Autodesk Fusion 360 part; units mm, degrees
note: some values were not read from the file. Chosen so that the rebuilt part matches the saved one: which face or edge a step refers to. Set by a fixed rule: which sketch regions a step uses.
(part 3 of 4)
sketch "Sketch5 (5)" plane through (0, 24.0807, 0) normal (0, 1, 0) x (-1, 0, 0) in component "ButtonRed v5"
  circle A0 centre (80.5, -16.1) radius 2.1574
  circle A1 centre (80.5, 16.1) radius 2.1574
  circle A2 centre (-80.5, -16.1) radius 2.1574
  circle A3 centre (-80.5, 16.1) radius 2.1574
  line L0 (-81.5, -11.1) -> (-83.5, -11.1)
  line L1 (-83.5, -11.1) -> (-83.5, -19.1)
  line L2 (-83.5, -19.1) -> (-75.5, -19.1)
  line L3 (-75.5, -19.1) -> (-75.5, -17.1)
  line L4 (-75.5, -17.1) -> (-45.2, -17.1)
  line L5 (-45.2, -17.1) -> (-45.2, -19.1)
  line L6 (-45.2, -19.1) -> (-37.2, -19.1)
  line L7 (-37.2, -19.1) -> (-37.2, -17.1)
  line L8 (-37.2, -17.1) -> (-4, -17.1)
  line L9 (-4, -17.1) -> (-4, -19.1)
  line L10 (-4, -19.1) -> (4, -19.1)
  line L11 (4, -19.1) -> (4, -17.1)
  line L12 (4, -17.1) -> (37.2, -17.1)
  line L13 (37.2, -17.1) -> (37.2, -19.1)
  line L14 (37.2, -19.1) -> (45.2, -19.1)
  line L15 (45.2, -19.1) -> (45.2, -17.1)
  line L16 (45.2, -17.1) -> (75.5, -17.1)
  line L17 (75.5, -17.1) -> (75.5, -19.1)
  line L18 (75.5, -19.1) -> (83.5, -19.1)
  line L19 (83.5, -19.1) -> (83.5, -11.1)
  line L20 (83.5, -11.1) -> (81.5, -11.1)
  line L21 (81.5, -11.1) -> (81.5, 11.1)
  line L22 (81.5, 11.1) -> (83.5, 11.1)
  line L23 (83.5, 11.1) -> (83.5, 19.1)
  line L24 (83.5, 19.1) -> (75.5, 19.1)
  line L25 (75.5, 19.1) -> (75.5, 17.1)
  line L26 (75.5, 17.1) -> (45.2, 17.1)
  line L27 (45.2, 17.1) -> (45.2, 19.1)
  line L28 (45.2, 19.1) -> (37.2, 19.1)
  line L29 (37.2, 19.1) -> (37.2, 17.1)
  line L30 (37.2, 17.1) -> (4, 17.1)
  line L31 (4, 17.1) -> (4, 19.1)
  line L32 (4, 19.1) -> (-4, 19.1)
  line L33 (-4, 19.1) -> (-4, 17.1)
  line L34 (-4, 17.1) -> (-37.2, 17.1)
  line L35 (-37.2, 17.1) -> (-37.2, 19.1)
  line L36 (-37.2, 19.1) -> (-45.2, 19.1)
  line L37 (-45.2, 19.1) -> (-45.2, 17.1)
  line L38 (-45.2, 17.1) -> (-75.5, 17.1)
  line L39 (-75.5, 17.1) -> (-75.5, 19.1)
  line L40 (-75.5, 19.1) -> (-83.5, 19.1)
  line L41 (-83.5, 19.1) -> (-83.5, 11.1)
  line L42 (-83.5, 11.1) -> (-81.5, 11.1)
  line L43 (-81.5, 11.1) -> (-81.5, -11.1)
  line L44 (-1, -11.1) -> (-1, 11.1)
  line L45 (-1, 11.1) -> (1, 11.1)
  line L46 (1, 11.1) -> (1, -11.1)
  line L47 (1, -11.1) -> (-1, -11.1)
  line L48 (-42.2, -11.1) -> (-42.2, 11.1)
  line L49 (-42.2, 11.1) -> (-40.2, 11.1)
  line L50 (-40.2, 11.1) -> (-40.2, -11.1)
  line L51 (-40.2, -11.1) -> (-42.2, -11.1)
  circle A4 centre (-61.8, 12.9) radius 3.1
  circle A5 centre (-20.6, 12.9) radius 3.1
  circle A6 centre (36, 0) radius 3.1
  circle A7 centre (77.2, 0) radius 3.1
  circle A8 centre (61.8, -12.9) radius 3.1
  circle A9 centre (20.6, -12.9) radius 3.1
  circle A10 centre (-5.2, 0) radius 3.1
  circle A11 centre (-61.8, -12.9) radius 3.1
  circle A12 centre (-46.4, 0) radius 3.1
  circle A13 centre (-20.6, -12.9) radius 3.1
  circle A14 centre (20.6, 12.9) radius 3.1
  circle A15 centre (61.8, 12.9) radius 3.1
  circle A16 centre (46.4, 0) radius 3.1
  circle A17 centre (5.2, 0) radius 3.1
  circle A18 centre (-36, 0) radius 3.1
  circle A19 centre (-77.2, 0) radius 3.1
  line L52 (9.4, 8.7) -> (31.8, 8.7)
  line L53 (31.8, 8.7) -> (31.8, -8.7)
  line L54 (31.8, -8.7) -> (9.4, -8.7)
  line L55 (9.4, -8.7) -> (9.4, 8.7)
  line L56 (-31.8, 8.7) -> (-9.4, 8.7)
  line L57 (-9.4, 8.7) -> (-9.4, -8.7)
  line L58 (-9.4, -8.7) -> (-31.8, -8.7)
  line L59 (-31.8, -8.7) -> (-31.8, 8.7)
  line L60 (73, 8.7) -> (73, -8.7)
  line L61 (73, -8.7) -> (50.6, -8.7)
  line L62 (50.6, -8.7) -> (50.6, 8.7)
  line L63 (50.6, 8.7) -> (73, 8.7)
  line L64 (-73, 8.7) -> (-50.6, 8.7)
  line L65 (-50.6, 8.7) -> (-50.6, -8.7)
  line L66 (-50.6, -8.7) -> (-73, -8.7)
  line L67 (-73, -8.7) -> (-73, 8.7)
  line L68 (42.2, 11.1) -> (42.2, -11.1)
  line L69 (42.2, -11.1) -> (40.2, -11.1)
  line L70 (40.2, -11.1) -> (40.2, 11.1)
  line L71 (40.2, 11.1) -> (42.2, 11.1)
  circle A20 centre (20.6, 12.9) radius 3.1
  line L72 (-1, -11.1) -> (1, -11.1)
  line L73 (1, -11.1) -> (1, 11.1)
  line L74 (1, 11.1) -> (-1, 11.1)
  line L75 (-1, 11.1) -> (-1, -11.1)
  circle A21 centre (20.6, -12.9) radius 3.1
  line L76 (4, -19.1) -> (37.2, -19.1)
  line L77 (37.2, -19.1) -> (37.2, -17.1)
  line L78 (37.2, -17.1) -> (4, -17.1)
  line L79 (4, -17.1) -> (4, -19.1)
  line L80 (42.2, 11.1) -> (40.2, 11.1)
  line L81 (40.2, 11.1) -> (40.2, -11.1)
  line L82 (40.2, -11.1) -> (42.2, -11.1)
  line L83 (42.2, -11.1) -> (42.2, 11.1)
  line L84 (37.2, 19.1) -> (4, 19.1)
  line L85 (4, 19.1) -> (4, 17.1)
  line L86 (4, 17.1) -> (37.2, 17.1)
  line L87 (37.2, 17.1) -> (37.2, 19.1)
  line L88 (39.6, -16.8333) -> (1.6, -16.8333)
  line L89 (1.6, -16.8333) -> (1.6, 16.6667)
  line L90 (1.6, 16.6667) -> (39.6, 16.6667)
  line L91 (39.6, 16.6667) -> (39.6, -16.8333)
  line L92 (39.6, -16.8333) -> (1.6, 16.6667) construction
  line L93 (1.6, -16.8333) -> (39.6, 16.6667) construction
  point P0 (5.2, 0)
  point P1 (20.6, -12.9)
  point P2 (20.6, -0.0833)
  dimension "d849_2" = 38
  dimension "d850_2" = 33.5
  constraint perpendicular L88 L89
  constraint parallel L88 L90
  constraint parallel L89 L91
  constraint horizontal L88
  constraint coincident L92 P2
  constraint coincident L93 P2
  measures "d849_2" distance of L89.end L90.end
  measures "d850_2" distance of L88.end L89.end
extrude "Extrude5''''" [suppressed] in component "ButtonRed v5"
sketch "Sketch7 (4)" plane through (0, 24.0807, 0) normal (0, 1, 0) x (-1, 0, 0) in component "ButtonRed v5"
  circle A0 centre (20.6, -12.9) radius 3.1
  circle A1 centre (20.6, 12.9) radius 3.1
  circle A2 centre (5.2, 0) radius 3.1
  circle A3 centre (36, 0) radius 3.1
  line L0 (39.6, 16.6667) -> (1.6, 16.6667)
  line L1 (1.6, 16.6667) -> (1.6, -16.8333)
  line L2 (1.6, -16.8333) -> (39.6, -16.8333)
  line L3 (39.6, -16.8333) -> (39.6, 16.6667)
  line L4 (39.6, -16.8333) -> (1.6, -16.8333)
  line L5 (1.6, -16.8333) -> (1.6, 16.6667)
  line L6 (1.6, 16.6667) -> (39.6, 16.6667)
  line L7 (39.6, 16.6667) -> (39.6, -16.8333)
  dimension "d859_2" = 38
  constraint horizontal L4
  constraint vertical L5
  constraint horizontal L6
  constraint vertical L7
  constraint coincident L0.end L1.start
  constraint coincident L2.end L3.start
  measures "d859_2" distance of L2.end L1.end
extrude "Extrude7''" [suppressed] in component "ButtonRed v5"
sketch "Sketch8 (4)" plane through (0, 25.2807, 0) normal (0, 1, 0) x (-1, 0, 0) in component "ButtonRed v5"
  line L0 (39.6, 16.6667) -> (1.6, 16.6667)
  line L1 (1.6, 16.6667) -> (1.6, -16.8333)
  line L2 (1.6, -16.8333) -> (39.6, -16.8333)
  line L3 (39.6, -16.8333) -> (39.6, 16.6667)
  circle A0 centre (20.6, -0.0833) radius 14
  dimension "d862_2" = 19
  dimension "d863_2" = 16.75
  dimension "d864_2" = 28
  dimension "d865_2" = 38
  dimension "d866_2" = 33.5
  measures "d862_2" distance of L1 A0.centre
  measures "d863_2" distance of L0 A0.centre
  measures "d864_2" diameter of A0
  measures "d865_2" distance of L1.end L2.end
  measures "d866_2" distance of L0.start L2.end
extrude "Extrude8'''" [suppressed] in component "ButtonRed v5"
sketch "Sketch9 (4)" plane through (-1.6, 0, 0) normal (1, 0, 0) x (0, 0, -1) in component "ButtonRed v5"
  line L0 (-16.6667, 25.2807) -> (-16.6667, 22.2807)
  line L1 (-16.6667, 22.2807) -> (16.8333, 22.2807)
  line L2 (16.8333, 22.2807) -> (16.8333, 25.2807)
  line L3 (16.8333, 25.2807) -> (-16.6667, 25.2807)
other "Base Feature1''" in component "ButtonGreen v6"
sketch "Sketch1 (7)" plane through (0, 45, 0) normal (0, 1, 0) x (-1, 0, 0) in component "ButtonGreen v6"
  line L0 (-111.8498, 7.1011) -> (-111.8498, -10.2989)
  line L1 (-111.8498, -10.2989) -> (-134.2498, -10.2989)
  line L2 (-134.2498, -10.2989) -> (-134.2498, 7.1011)
  line L3 (-134.2498, 7.1011) -> (-111.8498, 7.1011)
  circle A0 centre (-138.4498, -1.5989) radius 3.1
  circle A1 centre (-123.0498, 11.3011) radius 3.1
  circle A2 centre (-123.0498, -14.4989) radius 3.1
  circle A3 centre (-107.6498, -1.5989) radius 3.1
  line L4 (-103.4498, -18.6989) -> (-103.4498, 15.5011)
  line L5 (-103.4498, 15.5011) -> (-142.6498, 15.5011)
  line L6 (-142.6498, 15.5011) -> (-142.6498, -18.6989)
  line L7 (-142.6498, -18.6989) -> (-103.4498, -18.6989)
  circle A4 centre (-138.4498, -1.5989) radius 3.1
  circle A5 centre (-123.0498, -14.4989) radius 3.1
  circle A6 centre (-107.6498, -1.5989) radius 3.1
  circle A7 centre (-123.0498, 11.3011) radius 3.1
  line L8 (-154.8498, 7.1011) -> (-154.8498, -10.2989)
  line L9 (-177.2498, -10.2989) -> (-177.2498, 7.1011)
  line L10 (-146.7095, 15.4507) -> (-185.4095, 15.5014)
  line L11 (-177.2498, 7.1011) -> (-154.8498, 7.1011)
  circle A8 centre (-166.0498, -14.4989) radius 3.1
  circle A9 centre (-181.4498, -1.5989) radius 3.1
  line L12 (-185.4095, 15.5014) -> (-185.4536, -18.1986)
  circle A10 centre (-181.4498, -1.5989) radius 3.1
  line L13 (-146.7537, -18.2493) -> (-146.7095, 15.4507)
  circle A11 centre (-166.0498, 11.3011) radius 3.1
  circle A12 centre (-166.0498, 11.3011) radius 3.1
  line L14 (-154.8498, -10.2989) -> (-177.2498, -10.2989)
  circle A13 centre (-150.6498, -1.5989) radius 3.1
  circle A14 centre (-150.6498, -1.5989) radius 3.1
  line L15 (-185.4536, -18.1986) -> (-146.7537, -18.2493)
  circle A15 centre (-166.0498, -14.4989) radius 3.1
  arc A16 (86.5, -27.2432) -> (86.5, -22.3568) centre (88.5, -24.8) ccw
  arc A17 (-86.5, -22.3568) -> (-86.5, -27.2432) centre (-88.5, -24.8) ccw
  line L16 (86.5, 29) -> (-86.5, 29)
  line L17 (-86.5, 29) -> (-86.5, 27.2432)
  line L18 (-86.5, -29) -> (86.5, -29)
  line L19 (86.5, -29) -> (86.5, -27.2432)
  arc A18 (86.5, 22.3568) -> (86.5, 27.2432) centre (88.5, 24.8) ccw
  arc A19 (-86.5, 27.2432) -> (-86.5, 22.3568) centre (-88.5, 24.8) ccw
  line L20 (-86.5, 22.3568) -> (-86.5, -22.3568)
  line L21 (-86.5, -27.2432) -> (-86.5, -29)
  line L22 (86.5, -22.3568) -> (86.5, 22.3568)
  line L23 (86.5, 27.2432) -> (86.5, 29)
  dimension "d623_1" = 39.2
  dimension "d624_1" = 38.7
  dimension "d625_1" = 33.7
  dimension "d921_1" = 0
  dimension "d922_1" = 0
  dimension "d923_1" = 0
  dimension "d924_1" = 0
  constraint perpendicular L12 L15
  constraint parallel L10 L15
  constraint parallel L12 L13
  measures "d623_1" distance of L4.start L6.end
  measures "d624_1" distance of L13.start L12.end
  measures "d625_1" vertical distance of L10.end L12.end
extrude "Extrude1'''''" [suppressed] in component "ButtonGreen v6"
sketch "Sketch2 (6)" plane through (0, 45, 0) normal (0, 1, 0) x (-1, 0, 0) in component "ButtonGreen v6"
  line L0 (-142.6498, -18.6989) -> (-103.4498, -18.6989)
  line L1 (-103.4498, -18.6989) -> (-103.4498, 15.5011)
  line L2 (-103.4498, 15.5011) -> (-142.6498, 15.5011)
  line L3 (-142.6498, 15.5011) -> (-142.6498, -18.6989)
extrude "Extrude2''''''" [suppressed] in component "ButtonGreen v6"
sketch "Sketch3 (6)" plane through (0, 49.8, 0) normal (0, 1, 0) x (-1, 0, 0) in component "ButtonGreen v6"
  line L0 (-142.6498, 15.5011) -> (-142.6498, -18.6989)
  line L1 (-142.6498, -18.6989) -> (-103.4498, -18.6989)
  line L2 (-103.4498, -18.6989) -> (-103.4498, 15.5011)
  line L3 (-103.4498, 15.5011) -> (-142.6498, 15.5011)
  circle A0 centre (-123.0498, -1.5989) radius 14
  dimension "d616_1" = 28
  dimension "d617_1" = 17.1
  dimension "d618_1" = 34.2
  dimension "d619_1" = 39.2
  dimension "d620_1" = 19.6
  measures "d616_1" diameter of A0
  measures "d617_1" distance of L1 A0.centre
  measures "d618_1" distance of L1 L3
  measures "d619_1" distance of L0 L2
  measures "d620_1" distance of L2 A0.centre
extrude "Extrude3'''''" [suppressed] in component "ButtonGreen v6"
sketch "Sketch4 (6)" plane through (0, 49.8, 0) normal (0, 1, 0) x (-1, 0, 0) in component "ButtonGreen v6"
  circle A0 centre (-123.0498, -1.5989) radius 14
  line L0 (-142.6498, 15.5011) -> (-142.6498, -18.6989)
  line L1 (-142.6498, -18.6989) -> (-103.4498, -18.6989)
  line L2 (-103.4498, -18.6989) -> (-103.4498, 15.5011)
  line L3 (-103.4498, 15.5011) -> (-142.6498, 15.5011)
  line L4 (-103.9498, 15.0011) -> (-142.1498, 15.0011)
  line L5 (-142.1498, 15.0011) -> (-142.1498, -18.1989)
  line L6 (-142.1498, -18.1989) -> (-103.9498, -18.1989)
  line L7 (-103.9498, -18.1989) -> (-103.9498, 15.0011)
  dimension "d627_1" = -0.5
extrude "Extrude4'''''" [suppressed] in component "ButtonGreen v6"
sketch "Sketch10 (4)" plane through (0, 37.0807, 0) normal (0, 1, 0) x (-1, 0, 0) in component "ButtonGreen v6"
  circle A0 centre (80.75, -16) radius 2.1574
  circle A1 centre (80.75, 16.2) radius 2.1574
  circle A2 centre (-80.25, -16) radius 2.1574
  circle A3 centre (-80.25, 16.2) radius 2.1574
  line L0 (-81.25, -11) -> (-83.25, -11)
  line L1 (-83.25, -11) -> (-83.25, -19)
  line L2 (-83.25, -19) -> (-75.25, -19)
  line L3 (-75.25, -19) -> (-75.25, -17)
  line L4 (-75.25, -17) -> (-44.95, -17)
  line L5 (-44.95, -17) -> (-44.95, -19)
  line L6 (-44.95, -19) -> (-36.95, -19)
  line L7 (-36.95, -19) -> (-36.95, -17)
  line L8 (-36.95, -17) -> (-3.75, -17)
  line L9 (-3.75, -17) -> (-3.75, -19)
  line L10 (-3.75, -19) -> (4.25, -19)
  line L11 (4.25, -19) -> (4.25, -17)
  line L12 (4.25, -17) -> (37.45, -17)
  line L13 (37.45, -17) -> (37.45, -19)
  line L14 (37.45, -19) -> (45.45, -19)
  line L15 (45.45, -19) -> (45.45, -17)
  line L16 (45.45, -17) -> (75.75, -17)
  line L17 (75.75, -17) -> (75.75, -19)
  line L18 (75.75, -19) -> (83.75, -19)
  line L19 (83.75, -19) -> (83.75, -11)
  line L20 (83.75, -11) -> (81.75, -11)
  line L21 (81.75, -11) -> (81.75, 11.2)
  line L22 (81.75, 11.2) -> (83.75, 11.2)
  line L23 (83.75, 11.2) -> (83.75, 19.2)
  line L24 (83.75, 19.2) -> (75.75, 19.2)
  line L25 (75.75, 19.2) -> (75.75, 17.2)
  line L26 (75.75, 17.2) -> (45.45, 17.2)
  line L27 (45.45, 17.2) -> (45.45, 19.2)
  line L28 (45.45, 19.2) -> (37.45, 19.2)
  line L29 (37.45, 19.2) -> (37.45, 17.2)
  line L30 (37.45, 17.2) -> (4.25, 17.2)
  line L31 (4.25, 17.2) -> (4.25, 19.2)
  line L32 (4.25, 19.2) -> (-3.75, 19.2)
  line L33 (-3.75, 19.2) -> (-3.75, 17.2)
  line L34 (-3.75, 17.2) -> (-36.95, 17.2)
  line L35 (-36.95, 17.2) -> (-36.95, 19.2)
  line L36 (-36.95, 19.2) -> (-44.95, 19.2)
  line L37 (-44.95, 19.2) -> (-44.95, 17.2)
  line L38 (-44.95, 17.2) -> (-75.25, 17.2)
  line L39 (-75.25, 17.2) -> (-75.25, 19.2)
  line L40 (-75.25, 19.2) -> (-83.25, 19.2)
  line L41 (-83.25, 19.2) -> (-83.25, 11.2)
  line L42 (-83.25, 11.2) -> (-81.25, 11.2)
  line L43 (-81.25, 11.2) -> (-81.25, -11)
  line L44 (-0.75, -11) -> (-0.75, 11.2)
  line L45 (-0.75, 11.2) -> (1.25, 11.2)
  line L46 (1.25, 11.2) -> (1.25, -11)
  line L47 (1.25, -11) -> (-0.75, -11)
  line L48 (-41.95, -11) -> (-41.95, 11.2)
  line L49 (-41.95, 11.2) -> (-39.95, 11.2)
  line L50 (-39.95, 11.2) -> (-39.95, -11)
  line L51 (-39.95, -11) -> (-41.95, -11)
  circle A4 centre (-61.55, 13) radius 3.1
  circle A5 centre (-20.35, 13) radius 3.1
  circle A6 centre (36.25, 0.1) radius 3.1
  circle A7 centre (77.45, 0.1) radius 3.1
  circle A8 centre (62.05, -12.8) radius 3.1
  circle A9 centre (20.85, -12.8) radius 3.1
  circle A10 centre (-4.95, 0.1) radius 3.1
  circle A11 centre (-61.55, -12.8) radius 3.1
  circle A12 centre (-46.15, 0.1) radius 3.1
  circle A13 centre (-20.35, -12.8) radius 3.1
  circle A14 centre (20.85, 13) radius 3.1
  circle A15 centre (62.05, 13) radius 3.1
  circle A16 centre (46.65, 0.1) radius 3.1
  circle A17 centre (5.45, 0.1) radius 3.1
  circle A18 centre (-35.75, 0.1) radius 3.1
  circle A19 centre (-76.95, 0.1) radius 3.1
  line L52 (9.65, 8.8) -> (32.05, 8.8)
  line L53 (32.05, 8.8) -> (32.05, -8.6)
  line L54 (32.05, -8.6) -> (9.65, -8.6)
  line L55 (9.65, -8.6) -> (9.65, 8.8)
  line L56 (-31.55, 8.8) -> (-9.15, 8.8)
  line L57 (-9.15, 8.8) -> (-9.15, -8.6)
  line L58 (-9.15, -8.6) -> (-31.55, -8.6)
  line L59 (-31.55, -8.6) -> (-31.55, 8.8)
  line L60 (73.25, 8.8) -> (73.25, -8.6)
  line L61 (73.25, -8.6) -> (50.85, -8.6)
  line L62 (50.85, -8.6) -> (50.85, 8.8)
  line L63 (50.85, 8.8) -> (73.25, 8.8)
  line L64 (-72.75, 8.8) -> (-50.35, 8.8)
  line L65 (-50.35, 8.8) -> (-50.35, -8.6)
  line L66 (-50.35, -8.6) -> (-72.75, -8.6)
  line L67 (-72.75, -8.6) -> (-72.75, 8.8)
  line L68 (42.45, 11.2) -> (42.45, -11)
  line L69 (42.45, -11) -> (40.45, -11)
  line L70 (40.45, -11) -> (40.45, 11.2)
  line L71 (40.45, 11.2) -> (42.45, 11.2)
  circle A20 centre (62.05, 13) radius 3.1
  circle A21 centre (46.65, 0.1) radius 3.1
  circle A22 centre (62.05, -12.8) radius 3.1
  circle A23 centre (77.45, 0.1) radius 3.1
sketch "Sketch5 (6)" plane through (0, 24.0807, 0) normal (0, 1, 0) x (-1, 0, 0) in component "ButtonGreen v6"
  circle A0 centre (80.5, -16.1) radius 2.1574
  circle A1 centre (80.5, 16.1) radius 2.1574
  circle A2 centre (-80.5, -16.1) radius 2.1574
  circle A3 centre (-80.5, 16.1) radius 2.1574
  line L0 (-81.5, -11.1) -> (-83.5, -11.1)
  line L1 (-83.5, -11.1) -> (-83.5, -19.1)
  line L2 (-83.5, -19.1) -> (-75.5, -19.1)
  line L3 (-75.5, -19.1) -> (-75.5, -17.1)
  line L4 (-75.5, -17.1) -> (-45.2, -17.1)
  line L5 (-45.2, -17.1) -> (-45.2, -19.1)
  line L6 (-45.2, -19.1) -> (-37.2, -19.1)
  line L7 (-37.2, -19.1) -> (-37.2, -17.1)
  line L8 (-37.2, -17.1) -> (-4, -17.1)
  line L9 (-4, -17.1) -> (-4, -19.1)
  line L10 (-4, -19.1) -> (4, -19.1)
  line L11 (4, -19.1) -> (4, -17.1)
  line L12 (4, -17.1) -> (37.2, -17.1)
  line L13 (37.2, -17.1) -> (37.2, -19.1)
  line L14 (37.2, -19.1) -> (45.2, -19.1)
  line L15 (45.2, -19.1) -> (45.2, -17.1)
  line L16 (45.2, -17.1) -> (75.5, -17.1)
  line L17 (75.5, -17.1) -> (75.5, -19.1)
  line L18 (75.5, -19.1) -> (83.5, -19.1)
  line L19 (83.5, -19.1) -> (83.5, -11.1)
  line L20 (83.5, -11.1) -> (81.5, -11.1)
  line L21 (81.5, -11.1) -> (81.5, 11.1)
  line L22 (81.5, 11.1) -> (83.5, 11.1)
  line L23 (83.5, 11.1) -> (83.5, 19.1)
  line L24 (83.5, 19.1) -> (75.5, 19.1)
  line L25 (75.5, 19.1) -> (75.5, 17.1)
  line L26 (75.5, 17.1) -> (45.2, 17.1)
  line L27 (45.2, 17.1) -> (45.2, 19.1)
  line L28 (45.2, 19.1) -> (37.2, 19.1)
  line L29 (37.2, 19.1) -> (37.2, 17.1)
  line L30 (37.2, 17.1) -> (4, 17.1)
  line L31 (4, 17.1) -> (4, 19.1)
  line L32 (4, 19.1) -> (-4, 19.1)
  line L33 (-4, 19.1) -> (-4, 17.1)
  line L34 (-4, 17.1) -> (-37.2, 17.1)
  line L35 (-37.2, 17.1) -> (-37.2, 19.1)
  line L36 (-37.2, 19.1) -> (-45.2, 19.1)
  line L37 (-45.2, 19.1) -> (-45.2, 17.1)
  line L38 (-45.2, 17.1) -> (-75.5, 17.1)
  line L39 (-75.5, 17.1) -> (-75.5, 19.1)
  line L40 (-75.5, 19.1) -> (-83.5, 19.1)
  line L41 (-83.5, 19.1) -> (-83.5, 11.1)
  line L42 (-83.5, 11.1) -> (-81.5, 11.1)
  line L43 (-81.5, 11.1) -> (-81.5, -11.1)
  line L44 (-1, -11.1) -> (-1, 11.1)
  line L45 (-1, 11.1) -> (1, 11.1)
  line L46 (1, 11.1) -> (1, -11.1)
  line L47 (1, -11.1) -> (-1, -11.1)
  line L48 (-42.2, -11.1) -> (-42.2, 11.1)
  line L49 (-42.2, 11.1) -> (-40.2, 11.1)
  line L50 (-40.2, 11.1) -> (-40.2, -11.1)
  line L51 (-40.2, -11.1) -> (-42.2, -11.1)
  circle A4 centre (-61.8, 12.9) radius 3.1
  circle A5 centre (-20.6, 12.9) radius 3.1
  circle A6 centre (36, 0) radius 3.1
  circle A7 centre (77.2, 0) radius 3.1
  circle A8 centre (61.8, -12.9) radius 3.1
  circle A9 centre (20.6, -12.9) radius 3.1
  circle A10 centre (-5.2, 0) radius 3.1
  circle A11 centre (-61.8, -12.9) radius 3.1
  circle A12 centre (-46.4, 0) radius 3.1
  circle A13 centre (-20.6, -12.9) radius 3.1
  circle A14 centre (20.6, 12.9) radius 3.1
  circle A15 centre (61.8, 12.9) radius 3.1
  circle A16 centre (46.4, 0) radius 3.1
  circle A17 centre (5.2, 0) radius 3.1
  circle A18 centre (-36, 0) radius 3.1
  circle A19 centre (-77.2, 0) radius 3.1
  line L52 (9.4, 8.7) -> (31.8, 8.7)
  line L53 (31.8, 8.7) -> (31.8, -8.7)
  line L54 (31.8, -8.7) -> (9.4, -8.7)
  line L55 (9.4, -8.7) -> (9.4, 8.7)
  line L56 (-31.8, 8.7) -> (-9.4, 8.7)
  line L57 (-9.4, 8.7) -> (-9.4, -8.7)
  line L58 (-9.4, -8.7) -> (-31.8, -8.7)
  line L59 (-31.8, -8.7) -> (-31.8, 8.7)
  line L60 (73, 8.7) -> (73, -8.7)
  line L61 (73, -8.7) -> (50.6, -8.7)
  line L62 (50.6, -8.7) -> (50.6, 8.7)
  line L63 (50.6, 8.7) -> (73, 8.7)
  line L64 (-73, 8.7) -> (-50.6, 8.7)
  line L65 (-50.6, 8.7) -> (-50.6, -8.7)
  line L66 (-50.6, -8.7) -> (-73, -8.7)
  line L67 (-73, -8.7) -> (-73, 8.7)
  line L68 (42.2, 11.1) -> (42.2, -11.1)
  line L69 (42.2, -11.1) -> (40.2, -11.1)
  line L70 (40.2, -11.1) -> (40.2, 11.1)
  line L71 (40.2, 11.1) -> (42.2, 11.1)
  circle A20 centre (20.6, 12.9) radius 3.1
  line L72 (-1, -11.1) -> (1, -11.1)
  line L73 (1, -11.1) -> (1, 11.1)
  line L74 (1, 11.1) -> (-1, 11.1)
  line L75 (-1, 11.1) -> (-1, -11.1)
  circle A21 centre (20.6, -12.9) radius 3.1
  line L76 (4, -19.1) -> (37.2, -19.1)
  line L77 (37.2, -19.1) -> (37.2, -17.1)
  line L78 (37.2, -17.1) -> (4, -17.1)
  line L79 (4, -17.1) -> (4, -19.1)
  line L80 (42.2, 11.1) -> (40.2, 11.1)
  line L81 (40.2, 11.1) -> (40.2, -11.1)
  line L82 (40.2, -11.1) -> (42.2, -11.1)
  line L83 (42.2, -11.1) -> (42.2, 11.1)
  line L84 (37.2, 19.1) -> (4, 19.1)
  line L85 (4, 19.1) -> (4, 17.1)
  line L86 (4, 17.1) -> (37.2, 17.1)
  line L87 (37.2, 17.1) -> (37.2, 19.1)
  line L88 (39.6, -16.8333) -> (1.6, -16.8333)
  line L89 (1.6, -16.8333) -> (1.6, 16.6667)
  line L90 (1.6, 16.6667) -> (39.6, 16.6667)
  line L91 (39.6, 16.6667) -> (39.6, -16.8333)
  line L92 (39.6, -16.8333) -> (1.6, 16.6667) construction
  line L93 (1.6, -16.8333) -> (39.6, 16.6667) construction
  point P0 (5.2, 0)
  point P1 (20.6, -12.9)
  point P2 (20.6, -0.0833)
  dimension "d849_1" = 38
  dimension "d850_1" = 33.5
  constraint perpendicular L88 L89
  constraint parallel L88 L90
  constraint parallel L89 L91
  constraint horizontal L88
  constraint coincident L92 P2
  constraint coincident L93 P2
  measures "d849_1" distance of L89.end L90.end
  measures "d850_1" distance of L88.end L89.end
extrude "Extrude5'''''" [suppressed] in component "ButtonGreen v6"
sketch "Sketch7 (5)" plane through (0, 24.0807, 0) normal (0, 1, 0) x (-1, 0, 0) in component "ButtonGreen v6"
  circle A0 centre (20.6, -12.9) radius 3.1
  circle A1 centre (20.6, 12.9) radius 3.1
  circle A2 centre (5.2, 0) radius 3.1
  circle A3 centre (36, 0) radius 3.1
  line L0 (39.6, 16.6667) -> (1.6, 16.6667)
  line L1 (1.6, 16.6667) -> (1.6, -16.8333)
  line L2 (1.6, -16.8333) -> (39.6, -16.8333)
  line L3 (39.6, -16.8333) -> (39.6, 16.6667)
  line L4 (39.6, -16.8333) -> (1.6, -16.8333)
  line L5 (1.6, -16.8333) -> (1.6, 16.6667)
  line L6 (1.6, 16.6667) -> (39.6, 16.6667)
  line L7 (39.6, 16.6667) -> (39.6, -16.8333)
  dimension "d859_1" = 38
  constraint horizontal L4
  constraint vertical L5
  constraint horizontal L6
  constraint vertical L7
  constraint coincident L0.end L1.start
  constraint coincident L2.end L3.start
  measures "d859_1" distance of L2.end L1.end
extrude "Extrude7'''" [suppressed] in component "ButtonGreen v6"
sketch "Sketch8 (5)" plane through (0, 25.2807, 0) normal (0, 1, 0) x (-1, 0, 0) in component "ButtonGreen v6"
  line L0 (39.6, 16.6667) -> (1.6, 16.6667)
  line L1 (1.6, 16.6667) -> (1.6, -16.8333)
  line L2 (1.6, -16.8333) -> (39.6, -16.8333)
  line L3 (39.6, -16.8333) -> (39.6, 16.6667)
  circle A0 centre (20.6, -0.0833) radius 14
  dimension "d862_1" = 19
  dimension "d863_1" = 16.75
  dimension "d864_1" = 28
  dimension "d865_1" = 38
  dimension "d866_1" = 33.5
  measures "d862_1" distance of L1 A0.centre
  measures "d863_1" distance of L0 A0.centre
  measures "d864_1" diameter of A0
  measures "d865_1" distance of L1.end L2.end
  measures "d866_1" distance of L0.start L2.end
extrude "Extrude8''''" [suppressed] in component "ButtonGreen v6"
sketch "Sketch9 (5)" plane through (-1.6, 0, 0) normal (1, 0, 0) x (0, 0, -1) in component "ButtonGreen v6"
  line L0 (-16.6667, 25.2807) -> (-16.6667, 22.2807)
  line L1 (-16.6667, 22.2807) -> (16.8333, 22.2807)
  line L2 (16.8333, 22.2807) -> (16.8333, 25.2807)
  line L3 (16.8333, 25.2807) -> (-16.6667, 25.2807)
move_body "Move1" [suppressed] in component "Lid"
move_body "Move2" [suppressed] in component "Lid"
sketch "Sketch3 (7)" plane through (2.9698, 38.25, 1.2374) normal (0, 1, 0) x (-1, 0, 0) in component "Lid"
  line L0 (-61.7802, 11.7626) -> (125.7198, 11.7626)
  line L1 (125.7198, 11.7626) -> (125.7198, 69.7626)
  line L2 (-61.7802, 69.7626) -> (-61.7802, 11.7626)
  circle A0 centre (120.7198, 15.9626) radius 2
  circle A1 centre (120.7198, 65.5626) radius 2
  circle A2 centre (-56.7802, 15.9626) radius 2
  circle A3 centre (-56.7802, 65.5626) radius 2
  line L3 (125.7198, 69.7626) -> (-61.7802, 69.7626)
  dimension "d1030" = 4
  dimension "d1031" = 4.2
  dimension "d1033" = 187.5
  dimension "d1034" = 5
  dimension "d1035" = 5
  dimension "d1036" = 5
  dimension "d1037" = 4.2
  dimension "d1039" = 5
  constraint equal A0 A1
  constraint equal A0 A2
  constraint equal A0 A3
  measures "d1030" diameter of A0
  measures "d1031" distance of L0 A0.centre
  measures "d1033" distance of L0.start L0.end
  measures "d1034" distance of L1 A0.centre
  measures "d1035" distance of L1 A1.centre
  measures "d1036" distance of L2 A2.centre
  measures "d1037" distance of L0 A2.centre
  measures "d1039" distance of L2 A3.centre
extrude "Extrude3''''''" [suppressed] in component "Lid"
sketch "Sketch4 (7)" plane through (0, 38.25, 0) normal (0, 1, 0) x (-1, 0, 0) in component "Lid"
  line L0 (-64.75, 13) -> (122.75, 13)
  line L1 (122.75, 13) -> (122.75, 71)
  line L2 (-64.75, 71) -> (-64.75, 13)
  circle A0 centre (90.75, 43) radius 14.6
  line L3 (29, -29.0713) -> (29, 92.7233) construction
  line L4 (122.75, 71) -> (-64.75, 71)
  line L5 (-109.5632, 43) -> (-107.2358, 43)
  line L6 (-107.2358, 43) -> (154.5479, 43) construction
  circle A1 centre (49.55, 43) radius 14.6
  circle A2 centre (8.35, 43) radius 14.6
  circle A3 centre (-32.85, 43) radius 14.6
  circle A4 centre (117.75, 66.8) radius 2
  circle A5 centre (-59.75, 17.2) radius 2
  circle A6 centre (117.75, 17.2) radius 2
  circle A7 centre (-59.75, 66.8) radius 2
  line L7 (122.75, 71) -> (-64.75, 71)
  point P0 (29.9318, 42.6875)
  dimension "d1045" = 58
  dimension "d1053" = 29.2
  dimension "d1060" = 93.75
  dimension "d1061" = 187.5
  dimension "d1062" = 58
  dimension "d1064" = 30
  dimension "d1069" = 41.2
  dimension "d1070" = 41.2
  dimension "d1071" = 41.2
  dimension "d1085" = 32
  constraint vertical L3
  constraint horizontal L5
  constraint equal A0 A1
  constraint equal A1 A2
  constraint equal A2 A3
  constraint coincident A0.centre L6
  measures "d1045" distance of L0.start L2.start
  measures "d1053" diameter of A0
  measures "d1060" distance of L2 L3
  measures "d1061" distance of L1.end L2.start
  measures "d1062" distance of L0.start L2.start
  measures "d1064" distance of L0 L6
  measures "d1069" distance of A0.centre A1.centre
  measures "d1070" distance of A1.centre A2.centre
  measures "d1071" distance of A2.centre A3.centre
  measures "d1085" distance of L1 A0.centre
extrude "Extrude4''''''" [suppressed] in component "Lid"
sketch "Sketch16" plane through (0, 15, 0) normal (0, 1, 0) x (-1, 0, 0) in component "Button Base"
  line L0 (-4, 19.1) -> (-37.2, 19.1)
  line L1 (-37.2, 19.1) -> (-37.2, 17.1)
  line L2 (-37.2, 17.1) -> (-4, 17.1)
  line L3 (-4, 17.1) -> (-4, 19.1)
sketch "Sketch17" plane through (0, 0, 17.1) normal (0, 0, -1) x (-1, 0, 0) in component "Button Base"
  line L0 (-37.2, 7) -> (-4, 7)
  line L1 (-4, 7) -> (-4, 15)
  line L2 (-4, 15) -> (-37.2, 15)
  line L3 (-37.2, 15) -> (-37.2, 7)
ref_plane "WorkPlane3" through (40.2, 11, 0) normal (-1, 0, 0) x (0, 0, 1) in component "Button Base"
moveface "MoveFace1" [suppressed] in component "Button Base"
move_body "Move1'" [suppressed] in component "Button Base"
move_body "Move2'" [suppressed] in component "Button Base"
move_body "Move3" [suppressed] in component "Box"
move_body "Move3'" [suppressed] in component "Button Base"
ref_plane "WorkPlane1" through (-113.0665, 43.4789, -26.3874) normal (-1, 0, 0) x (0, 0, -1) in component "Component''"
sketch "Sketch4 (8)" plane through (0, 0, -66.2581) normal (0, 0, -1) x (-1, 0, 0)
  line L0 (21.2628, 41.0959) -> (194.7628, 41.0959)
  line L1 (194.7628, 41.0959) -> (194.7628, 74.0959)
  line L2 (194.7628, 74.0959) -> (21.2628, 74.0959)
  line L3 (21.2628, 74.0959) -> (21.2628, 41.0959)
sketch "Sketch8 (6)" plane through (0, 38.25, 0) normal (0, 1, 0) x (-1, 0, 0) in component "Lid"
  circle A0 centre (54.55, -2) radius 14.6
  circle A1 centre (13.35, -2) radius 14.6
  circle A2 centre (95.75, -2) radius 14.6
  circle A3 centre (-27.85, -2) radius 14.6
  line L0 (-59.75, -32) -> (127.75, -32)
  line L1 (127.75, -32) -> (127.75, 26)
  line L2 (-59.75, 26) -> (-59.75, -32)
  circle A4 centre (122.75, 21.8) radius 2
  circle A5 centre (-54.75, -27.8) radius 2
  circle A6 centre (122.75, -27.8) radius 2
  circle A7 centre (-54.75, 21.8) radius 2
  line L3 (127.75, 26) -> (-59.75, 26)
sketch "Sketch9 (6)" plane through (0, 38.25, 0) normal (0, 1, 0) x (-1, 0, 0) in component "Lid"
sketch "Sketch1 (8)" plane through (-190, 0, 2.6126) normal (0, 0, 1) x (1, 0, 0) in component "Component''"
  line L0 (150.6835, 28.4789) -> (-6.8165, 28.4789)
  line L1 (-6.8165, 58.4789) -> (-9.8165, 58.4789)
  line L2 (-9.8165, 58.4789) -> (-9.8165, 25.4789)
  line L3 (-9.8165, 25.4789) -> (163.6835, 25.4789)
  line L4 (-6.8165, 28.4789) -> (-6.8165, 20)
  line L5 (-6.8165, 20) -> (14.8335, 20)
  line L6 (14.8335, 20) -> (76.9209, 20)
  line L7 (76.9209, 20) -> (76.9209, 68.6959)
  line L8 (76.9209, 68.6959) -> (14.8335, 68.6959)
  line L9 (14.8335, 68.6959) -> (14.8335, 20)
  line L10 (163.6835, 25.4789) -> (163.6835, 58.4789)
  line L11 (163.6835, 58.4789) -> (150.6835, 58.4789)
  line L12 (150.6835, 58.4789) -> (150.6835, 28.4789)
  line L13 (-6.8165, 28.4789) -> (-6.8165, 58.4789)
  dimension "d1323" = 21.65
  constraint coincident L0.end L4.start
  constraint perpendicular L3 L4
  constraint perpendicular L4 L5
  constraint horizontal L6
  constraint vertical L7
  constraint horizontal L8
  constraint vertical L9
  measures "d1323" distance of L4.end L5.end
sketch "Sketch2 (7)" plane through (-190, 0, 2.6126) normal (0, 0, 1) x (1, 0, 0) in component "Component''"
  line L0 (-9.8165, 25.4789) -> (163.6835, 25.4789)
  line L1 (163.6835, 25.4789) -> (163.6835, 58.4789)
  line L2 (-6.8165, 58.4789) -> (-9.8165, 58.4789)
  line L3 (150.6835, 28.4789) -> (-6.8165, 28.4789)
  line L4 (150.6835, 28.4789) -> (128.5335, 28.4789)
  line L5 (128.5335, 28.4789) -> (128.5335, 68)
  line L6 (128.5335, 68) -> (60, 68)
  line L7 (60, 68) -> (60, 24.8783)
  line L8 (60, 24.8783) -> (128.5335, 24.8783)
  line L9 (128.5335, 24.8783) -> (128.5335, 28.4789)
  line L10 (-9.8165, 58.4789) -> (-9.8165, 25.4789)
  line L11 (163.6835, 58.4789) -> (150.6835, 58.4789)
  line L12 (150.6835, 58.4789) -> (150.6835, 28.4789)
  line L13 (-6.8165, 28.4789) -> (-6.8165, 58.4789)
  dimension "d1328" = 22.15
  constraint coincident L3.start L4.start
  constraint perpendicular L4 L5
  constraint perpendicular L5 L6
  constraint perpendicular L6 L7
  constraint perpendicular L7 L8
  constraint perpendicular L8 L9
  measures "d1328" distance of L3.start L4.end
sketch "Sketch3 (8)" plane through (-190, 0, 2.6126) normal (0, 0, 1) x (1, 0, 0) in component "Component''"
  line L0 (150.6835, 28.4789) -> (-6.8165, 28.4789)
  line L1 (-6.8165, 58.4789) -> (-9.8165, 58.4789)
  line L2 (-9.8165, 58.4789) -> (-9.8165, 25.4789)
  line L3 (-9.8165, 25.4789) -> (163.6835, 25.4789)
  line L4 (163.6835, 25.4789) -> (163.6835, 58.4789)
  line L5 (163.6835, 58.4789) -> (150.6835, 58.4789)
  line L6 (150.6835, 58.4789) -> (150.6835, 28.4789)
  line L7 (-6.8165, 28.4789) -> (-6.8165, 58.4789)
sketch "Sketch5 (7)" plane through (0, 0, 47.6126) normal (0, 0, 1) x (1, 0, 0) in component "Component''"
  line L0 (36.9372, 44.0959) -> (14.7872, 44.0959)
  line L1 (-1.8165, 28.4789) -> (-1.8165, 58.4789)
  line L2 (-1.8165, 58.4789) -> (-4.8165, 58.4789)
  line L3 (-4.8165, 58.4789) -> (-4.8165, 25.4789)
  line L4 (14.7872, 41.0959) -> (39.9372, 41.0959)
  line L5 (39.9372, 41.0959) -> (39.9372, 74.0959)
  line L6 (39.9372, 74.0959) -> (36.9372, 74.0959)
  line L7 (36.9372, 74.0959) -> (36.9372, 44.0959)
  line L8 (14.7872, 44.0959) -> (14.7872, 41.0959)
  line L9 (19.8335, 25.4789) -> (19.8335, 28.4789)
  line L10 (19.8335, 28.4789) -> (-1.8165, 28.4789)
  line L11 (-4.8165, 25.4789) -> (19.8335, 25.4789)
split "Split1" [suppressed] in component "Lid"
sketch "Sketch5 (8)" plane through (0, 0, 26) normal (0, 0, 1) x (1, 0, 0) in component "Lid"
  line L0 (59.75, 33) -> (59.75, 38.25)
  line L1 (-37.25, 38.8352) -> (51.75, 38.8352)
  line L2 (51.75, 38.8352) -> (51.75, 32.8352)
  line L3 (51.75, 32.8352) -> (-37.25, 32.8352)
  line L4 (-37.25, 32.8352) -> (-37.25, 38.8352)
  line L5 (-127.75, 38.25) -> (-127.75, 33)
  dimension "d1341" = 89
  dimension "d1342" = 6
  dimension "d1343" = 8
  constraint horizontal L1
  constraint vertical L2
  constraint horizontal L3
  constraint vertical L4
  measures "d1341" distance of L1.start L1.end
  measures "d1342" distance of L1.end L2.end
  measures "d1343" distance of L0 L2
extrude "Extrude5''''''" [suppressed] in component "Lid"
sketch "Sketch6 (2)" plane through (0, 0, 26) normal (0, 0, 1) x (1, 0, 0) in component "Lid"
  line L0 (59.75, 38.25) -> (-127.75, 38.25)
  line L1 (-127.75, 38.25) -> (-127.75, 33)
  line L2 (-127.75, 33) -> (59.75, 33)
  line L3 (-127.75, 35.625) -> (-127.75, 39.7713)
  line L4 (-127.75, 39.7713) -> (-76.75, 39.7713)
  line L5 (-76.75, 39.7713) -> (-33.2597, 39.7713)
  line L6 (-33.2597, 39.7713) -> (-33.2597, 32.3393)
  line L7 (-33.2597, 32.3393) -> (-76.75, 32.3393)
  line L8 (-76.75, 32.3393) -> (-76.75, 39.7713)
  line L9 (59.75, 33) -> (59.75, 38.25)
  dimension "d1346" = 51
  constraint midpoint L1 L3.start
  constraint perpendicular L0 L3
  constraint perpendicular L1 L4
  constraint horizontal L5
  constraint vertical L6
  constraint horizontal L7
  constraint vertical L8
  measures "d1346" distance of L3.end L4.end
extrude "Extrude6" [suppressed] in component "Lid"
sketch "Sketch7 (6)" plane through (0, 38.25, 0) normal (0, 1, 0) x (-1, 0, 0) in component "Lid"
  line L0 (-59.75, -32) -> (127.75, -32)
  line L1 (127.75, -32) -> (127.75, 26)
  circle A0 centre (95.75, -2) radius 14.6
  circle A1 centre (54.55, -2) radius 14.6
  line L2 (127.75, -32) -> (77.75, -32)
  line L3 (77.75, -32) -> (77.75, 26)
  line L4 (77.75, 26) -> (127.75, 26)
  line L5 (127.75, 26) -> (127.75, -32)
  line L6 (77.75, -32) -> (34, -32)
  line L7 (34, -32) -> (34, 26.2118)
  line L8 (34, 26.2118) -> (77.75, 26.2118)
  line L9 (77.75, 26.2118) -> (77.75, -32)
  circle A2 centre (13.35, -2) radius 14.6
  circle A3 centre (-27.85, -2) radius 14.6
  line L10 (-59.75, 26) -> (-59.75, -32)
  circle A4 centre (122.75, 21.8) radius 2
  circle A5 centre (-54.75, -27.8) radius 2
  circle A6 centre (122.75, -27.8) radius 2
  circle A7 centre (-54.75, 21.8) radius 2
  line L11 (127.75, 26) -> (-59.75, 26)
  dimension "d1349" = 50
  constraint horizontal L2
  constraint vertical L3
  constraint horizontal L4
  constraint vertical L5
  constraint coincident L0.end L1.start
  constraint horizontal L6
  constraint vertical L7
  constraint horizontal L8
  constraint vertical L9
  measures "d1349" distance of L0.end L2.end
extrude "Extrude7''''" [suppressed] in component "Lid"
move_body "Move3''" [suppressed] in component "Lid"
split "Split2" [suppressed] in component "Button"
sketch "Sketch11" plane through (0, 24.6807, 0) normal (0, -1, 0) x (1, 0, 0) in component "Button"
  circle A0 centre (-23.8871, 65.1319) radius 14
  circle A1 centre (-23.8871, 65.1319) radius 2.2005
  line L0 (-19.8871, 62.6319) -> (-27.8871, 62.6319)
  line L1 (-27.8871, 62.6319) -> (-27.8871, 67.6319)
  line L2 (-27.8871, 67.6319) -> (-19.8871, 67.6319)
  line L3 (-19.8871, 67.6319) -> (-19.8871, 62.6319)
  line L4 (-19.8871, 62.6319) -> (-27.8871, 67.6319) construction
  line L5 (-27.8871, 62.6319) -> (-19.8871, 67.6319) construction
  point P0 (-23.8871, 65.1319)
  dimension "d1543" = 8
  dimension "d1544" = 5
  constraint concentric A0 A1
  constraint perpendicular L0 L1
  constraint parallel L0 L2
  constraint parallel L1 L3
  constraint horizontal L0
  constraint coincident L4 P0
  constraint coincident L5 P0
  constraint coincident P0 A0.centre
  measures "d1543" distance of L1.end L2.end
  measures "d1544" distance of L0.start L2.end
extrude "Extrude11'" [suppressed] in component "Button"
sketch "Sketch12 (2)" plane through (0, 21.6807, 0) normal (0, -1, 0) x (1, 0, 0) in component "Button"
  circle A0 centre (-8.4871, 65.2152) radius 2.95
  circle A1 centre (-39.2871, 65.2152) radius 2.95
  circle A2 centre (-23.8871, 52.3152) radius 2.95
  circle A3 centre (-23.8871, 78.1152) radius 2.95
  line L0 (-4.8871, 81.8819) -> (-42.8871, 81.8819)
  line L1 (-42.8871, 81.8819) -> (-42.8871, 48.3819)
  line L2 (-42.8871, 48.3819) -> (-4.8871, 48.3819)
  line L3 (-4.8871, 48.3819) -> (-4.8871, 81.8819)
  line L4 (-19.4871, 62.2319) -> (-28.2871, 62.2319)
  line L5 (-28.2871, 62.2319) -> (-28.2871, 68.0319)
  line L6 (-28.2871, 68.0319) -> (-19.4871, 68.0319)
  line L7 (-19.4871, 68.0319) -> (-19.4871, 62.2319)
  line L8 (-19.4871, 62.2319) -> (-28.2871, 68.0319) construction
  line L9 (-28.2871, 62.2319) -> (-19.4871, 68.0319) construction
  line L10 (-4.8871, 81.8819) -> (-4.8871, 48.3819)
  point P0 (-23.8871, 65.1319)
  dimension "d1547" = 8.8
  dimension "d1548" = 5.8
  dimension "d1549" = 19
  dimension "d1550" = 16.75
  constraint perpendicular L4 L5
  constraint parallel L4 L6
  constraint parallel L5 L7
  constraint horizontal L4
  constraint coincident L8 P0
  constraint coincident L9 P0
  measures "d1547" distance of L5.end L6.end
  measures "d1548" distance of L4.start L6.end
  measures "d1549" distance of P0 L10
  measures "d1550" distance of L2 P0
sketch "Sketch13 (2)" plane through (0, 0, 48.3819) normal (0, 0, -1) x (-1, 0, 0) in component "Button"
  line L0 (4.8871, 24.6807) -> (4.8871, 21.6807)
  line L1 (4.8871, 21.6807) -> (42.8871, 21.6807)
  line L2 (42.8871, 21.6807) -> (42.8871, 24.6807)
  line L3 (42.8871, 24.6807) -> (4.8871, 24.6807)
sketch "Sketch14" plane through (0, 21.6807, 0) normal (0, -1, 0) x (1, 0, 0) in component "Button"
  circle A0 centre (-8.4871, 65.2152) radius 2.95
  circle A1 centre (-39.2871, 65.2152) radius 2.95
  circle A2 centre (-23.8871, 52.3152) radius 2.95
  circle A3 centre (-23.8871, 78.1152) radius 2.95
  line L0 (-4.8871, 81.8819) -> (-42.8871, 81.8819)
  line L1 (-42.8871, 81.8819) -> (-42.8871, 48.3819)
  line L2 (-42.8871, 48.3819) -> (-4.8871, 48.3819)
  line L3 (-4.8871, 48.3819) -> (-4.8871, 81.8819)
  line L4 (-19.4871, 62.2319) -> (-28.2871, 62.2319)
  line L5 (-28.2871, 62.2319) -> (-28.2871, 68.0319)
  line L6 (-28.2871, 68.0319) -> (-19.4871, 68.0319)
  line L7 (-19.4871, 68.0319) -> (-19.4871, 62.2319)
  line L8 (-19.4871, 62.2319) -> (-28.2871, 68.0319) construction
  line L9 (-28.2871, 62.2319) -> (-19.4871, 68.0319) construction
  line L10 (-4.8871, 81.8819) -> (-4.8871, 48.3819)
  point P0 (-23.8871, 65.1319)
  dimension "d1553" = 8.8
  dimension "d1554" = 5.8
  dimension "d1555" = 19
  dimension "d1557" = 16.75
  constraint perpendicular L4 L5
  constraint parallel L4 L6
  constraint parallel L5 L7
  constraint horizontal L4
  constraint coincident L8 P0
  constraint coincident L9 P0
  measures "d1553" distance of L5.end L6.end
  measures "d1554" distance of L4.start L6.end
  measures "d1555" distance of P0 L10
  measures "d1557" distance of L0 P0
extrude "Extrude13" [suppressed] in component "Button"
split "Split1'" [suppressed] in component "Button"
sketch "Sketch1 (9)" plane through (-185.2281, 69.0959, -11.0155) normal (0, 1, 0) x (-1, 0, 0)
  line L0 (-80.5653, 2.0074) -> (-42.5653, 2.0074)
  line L1 (-42.5653, 2.0074) -> (-42.5653, 35.5074)
  line L2 (-42.5653, 35.5074) -> (-80.5653, 35.5074)
  line L3 (-80.5653, 35.5074) -> (-80.5653, 2.0074)
  circle A0 centre (-61.5653, 18.7574) radius 14
  line L4 (-42.5653, 35.5074) -> (-42.5653, 2.0074)
  line L5 (-60.0653, 17.2574) -> (-63.0653, 17.2574)
  line L6 (-63.0653, 17.2574) -> (-63.0653, 20.2574)
  line L7 (-63.0653, 20.2574) -> (-60.0653, 20.2574)
  line L8 (-60.0653, 20.2574) -> (-60.0653, 17.2574)
  line L9 (-60.0653, 17.2574) -> (-63.0653, 20.2574) construction
  line L10 (-63.0653, 17.2574) -> (-60.0653, 20.2574) construction
  line L11 (42.8871, 81.8819) -> (4.8871, 81.8819)
  line L12 (4.8871, 81.8819) -> (4.8871, 48.3819)
  line L13 (4.8871, 48.3819) -> (42.8871, 48.3819)
  line L14 (42.8871, 48.3819) -> (42.8871, 81.8819)
  line L15 (-80.5653, 2.0074) -> (-42.5653, 2.0074)
  line L16 (-42.5653, 2.0074) -> (-42.5653, 35.5074)
  line L17 (-42.5653, 35.5074) -> (-80.5653, 35.5074)
  line L18 (-80.5653, 35.5074) -> (-80.5653, 2.0074)
  line L19 (-57.1653, 21.6574) -> (-57.1653, 15.8574)
  line L20 (-57.1653, 15.8574) -> (-65.9653, 15.8574)
  line L21 (-65.9653, 15.8574) -> (-65.9653, 21.6574)
  line L22 (-65.9653, 21.6574) -> (-57.1653, 21.6574)
  point P0 (-61.5653, 18.7574)
  dimension "d1475" = 28
  dimension "d1476" = 19
  dimension "d1477" = 16.75
  dimension "d1478" = 3
  dimension "d1479" = 3
  dimension "d1480" = 1.5
  constraint perpendicular L5 L6
  constraint parallel L5 L7
  constraint parallel L6 L8
  constraint horizontal L5
  constraint coincident L9 P0
  constraint coincident L10 P0
  constraint coincident P0 A0.centre
  measures "d1475" diameter of A0
  measures "d1476" distance of P0 L4
  measures "d1477" distance of L0 P0
  measures "d1478" distance of L6.end L7.end
  measures "d1479" distance of L5.end L6.end
  measures "d1480" distance of L8 P0
extrude "Extrude9''" [suppressed] in component "Button"
sketch "Sketch2 (8)" plane through (-185.2281, 10.617, 24.4919) normal (0, 0, 1) x (1, 0, 0)
  line L0 (42.5653, 58.4789) -> (42.5653, 55.4789)
  line L1 (42.5653, 55.4789) -> (80.5653, 55.4789)
  line L2 (80.5653, 55.4789) -> (80.5653, 58.4789)
  line L3 (80.5653, 58.4789) -> (42.5653, 58.4789)
sketch "Sketch3 (9)" plane through (-185.2281, 69.0959, -11.0155) normal (0, -1, 0) x (1, 0, 0)
  circle A0 centre (61.5653, 18.7574) radius 14
  circle A1 centre (61.5653, 18.7574) radius 10.5988
  line L0 (60.2653, 20.0574) -> (62.8653, 20.0574)
  line L1 (62.8653, 20.0574) -> (62.8653, 17.4574)
  line L2 (62.8653, 17.4574) -> (60.2653, 17.4574)
  line L3 (60.2653, 17.4574) -> (60.2653, 20.0574)
  line L4 (60.2653, 20.0574) -> (62.8653, 17.4574) construction
  line L5 (62.8653, 20.0574) -> (60.2653, 17.4574) construction
  line L6 (75.5653, 4.7574) -> (47.5653, 4.7574)
  line L7 (47.5653, 4.7574) -> (47.5653, 32.7574)
  line L8 (47.5653, 32.7574) -> (75.5653, 32.7574)
  line L9 (75.5653, 32.7574) -> (75.5653, 4.7574)
  point P0 (61.5653, 18.7574)
  dimension "d1483" = 2.6
  dimension "d1484" = 2.6
  dimension "d1485" = 28
  dimension "d1486" = 28
  dimension "d1487" = 14
  dimension "d1488" = 14
  constraint concentric A0 A1
  constraint perpendicular L0 L1
  constraint parallel L0 L2
  constraint parallel L1 L3
  constraint horizontal L0
  constraint coincident L4 P0
  constraint coincident L5 P0
  constraint coincident P0 A0.centre
  constraint horizontal L6
  constraint vertical L7
  constraint horizontal L8
  constraint vertical L9
  measures "d1483" distance of L1.end L2.end
  measures "d1484" distance of L0.start L2.end
  measures "d1485" distance of L6.start L6.end
  measures "d1486" distance of L6.start L8.end
  measures "d1487" distance of P0 L7
  measures "d1488" distance of P0 L8
extrude "Extrude10'" [suppressed] in component "Button"
sketch "Sketch5 (9)" plane through (-24.6645, 15.1624, 5.2419) normal (0, 0, -1) x (-1, 0, 0)
  line L0 (102.9983, 53.9335) -> (94.9983, 53.9335)
  line L1 (94.9983, 53.9335) -> (94.9983, 46.9335)
  line L2 (94.9983, 46.9335) -> (102.9983, 46.9335)
  line L3 (102.9983, 46.9335) -> (102.9983, 53.9335)
sketch "Sketch6 (3)" plane through (-24.6645, 15.1624, 10.2419) normal (0, 0, 1) x (1, 0, 0)
  line L0 (-94.9983, 53.9335) -> (-102.9983, 53.9335)
  line L1 (-102.9983, 53.9335) -> (-102.9983, 46.9335)
  line L2 (-102.9983, 46.9335) -> (-94.9983, 46.9335)
  line L3 (-94.9983, 46.9335) -> (-94.9983, 53.9335)
sketch "Sketch10 (5)" plane through (-34.15, 38.25, -2.3) normal (0, 1, 0) x (1, 0, 0) in component "Lid"
  circle A0 centre (27.85, -2) radius 14.6
  circle A1 centre (54.75, -27.8) radius 3.05
  circle A2 centre (54.75, 21.8) radius 3.05
  line L0 (59.75, -32) -> (59.75, 26)
  line L1 (-76.3, -20.05) -> (-115.6, -20.05)
  line L2 (-115.6, -20.05) -> (-115.6, 14.05)
  line L3 (-115.6, 14.05) -> (-76.3, 14.05)
  line L4 (-76.3, 14.05) -> (-76.3, -20.05)
  line L5 (-76.3, -20.05) -> (-115.6, 14.05)
  line L6 (-115.6, -20.05) -> (-76.3, 14.05)
  line L7 (-210, -3) -> (63.2922, -3) construction
  line L8 (-34, 80) -> (-34, -63.8009) construction
  line L9 (59.75, 26) -> (-127.75, 26)
  line L10 (-127.75, -32) -> (59.75, -32)
  line L11 (-35, -20.05) -> (-74.3, -20.05)
  line L12 (-74.3, -20.05) -> (-74.3, 14.05)
  line L13 (-74.3, 14.05) -> (-35, 14.05)
  line L14 (-35, 14.05) -> (-35, -20.05)
  line L15 (-35, -20.05) -> (-74.3, 14.05) construction
  line L16 (-74.3, -20.05) -> (-35, 14.05) construction
  line L17 (6.3, -19.05) -> (-33, 15.05) construction
  line L18 (6.3, -19.05) -> (-33, -19.05)
  line L19 (6.3, 15.05) -> (6.3, -19.05)
  line L20 (-33, -19.05) -> (-33, 15.05)
  line L21 (-33, -19.05) -> (6.3, 15.05) construction
  line L22 (-33, 15.05) -> (6.3, 15.05)
  line L23 (47.6, -20.05) -> (8.3, 14.05) construction
  line L24 (47.6, -20.05) -> (8.3, -20.05)
  line L25 (47.6, 14.05) -> (47.6, -20.05)
  line L26 (8.3, -20.05) -> (8.3, 14.05)
  line L27 (8.3, -20.05) -> (47.6, 14.05) construction
  line L28 (8.3, 14.05) -> (47.6, 14.05)
  line L29 (-127.75, 26) -> (-127.75, -32)
  line L30 (83.5, -3) -> (-83.5, -3)
  line L31 (-83.5, -3) -> (-83.5, -7)
  line L32 (-83.5, -7) -> (-75.5, -7)
  line L33 (-75.5, -7) -> (-75.5, -15)
  line L34 (-75.5, -15) -> (-45.2, -15)
  line L35 (-45.2, -15) -> (-45.2, -7)
  line L36 (-45.2, -7) -> (-37.2, -7)
  line L37 (-37.2, -7) -> (-37.2, -15)
  line L38 (-37.2, -15) -> (-4, -15)
  line L39 (-4, -15) -> (-4, -7)
  line L40 (-4, -7) -> (4, -7)
  line L41 (4, -7) -> (4, -15)
  line L42 (4, -15) -> (37.2, -15)
  line L43 (37.2, -15) -> (37.2, -7)
  line L44 (37.2, -7) -> (45.2, -7)
  line L45 (45.2, -7) -> (45.2, -15)
  line L46 (45.2, -15) -> (75.5, -15)
  line L47 (75.5, -15) -> (75.5, -7)
  line L48 (75.5, -7) -> (83.5, -7)
  line L49 (83.5, -7) -> (83.5, -3)
  line L50 (37.2, 19.1) -> (4, 19.1)
  line L51 (4, 19.1) -> (4, 17.1)
  line L52 (4, 17.1) -> (37.2, 17.1)
  line L53 (37.2, 17.1) -> (37.2, 19.1)
  circle A3 centre (-20.4, -0.3) radius 14.6
  circle A4 centre (20.8, -0.3) radius 14.6
  circle A5 centre (-61.6, -0.3) radius 14.6
  circle A6 centre (62, -0.3) radius 14.6
  line L54 (93.9, 29.7) -> (-93.6, 29.7)
  line L55 (-93.6, 29.7) -> (-93.6, -28.3)
  line L56 (93.9, -28.3) -> (93.9, 29.7)
  circle A7 centre (-88.6, -24.1) radius 2
  circle A8 centre (88.9, 25.5) radius 2
  circle A9 centre (-88.6, 25.5) radius 2
  circle A10 centre (88.9, -24.1) radius 2
  line L57 (-93.6, -28.3) -> (93.9, -28.3)
  point P0 (-95.95, -3)
  point P1 (-54.65, -3)
  point P2 (-13.35, -2)
  point P3 (27.95, -3)
  dimension "d1594" = 39.3
  dimension "d1595" = 34.1
  dimension "d1596" = 93.75
  dimension "d1597" = 29
  dimension "d1598" = 58
  dimension "d1600" = 2
  dimension "d1601" = 2
  dimension "d1602" = 2
  dimension "d1608" = 1
  dimension "d1609" = 30
  dimension "d1610" = 29
  constraint perpendicular L1 L2
  constraint parallel L1 L3
  constraint parallel L2 L4
  constraint horizontal L1
  constraint coincident L5 P0
  constraint coincident L6 P0
  constraint perpendicular L0 L7
  constraint vertical L8
  constraint coincident P0 L7
  constraint perpendicular L11 L12
  constraint parallel L11 L13
  constraint parallel L12 L14
  constraint horizontal L11
  constraint coincident L15 P1
  constraint coincident L16 P1
  constraint coincident L7 P1
  constraint equal L3 L13
  constraint equal L4 L12
  constraint perpendicular L18 L20
  constraint parallel L18 L22
  constraint parallel L19 L20
  constraint horizontal L18
  constraint coincident P2 L17
  constraint coincident P2 L21
  constraint perpendicular L24 L26
  constraint parallel L24 L28
  constraint parallel L25 L26
  constraint horizontal L24
  constraint coincident P3 L23
  constraint coincident P3 L27
  constraint equal L13 L22
  constraint equal L13 L28
  constraint equal L2 L20
  constraint equal L2 L26
  measures "d1594" distance of L2.end L3.end
  measures "d1595" distance of L1.end L2.end
  measures "d1596" distance of L0 L8
  measures "d1597" distance of L7 L9
  measures "d1598" distance of L9 L10
  measures "d1600" distance of L4 L12
  measures "d1601" distance of L14 L20
  measures "d1602" distance of L19 L26
  measures "d1608" distance of L8 L14
  measures "d1609" distance of L10 P2
  measures "d1610" distance of L10 P3